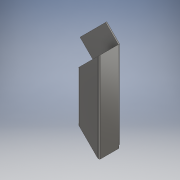
# Autodesk Inventor part: TestPlate
Saved by Autodesk Inventor 2018 (Build 220112000, 112)
## iProperties
Created: 2018-02-27
Part Number: TestPlate
Material: Steel, Mild
Document SubType Name: Modeling
Designer: P136265
Density: 7.85 g/cm^3
Appearance: Semi-Polished
Mass: 466.656 g
Surface Area: 399.113 cm^2
Volume: 59.4467 cm^3
Author: P136265
Autodesk Inventor part; units mm, degrees
ref_plane "YZ Plane" through (0, 0, 0) normal (1, 0, 0) x (0, 1, 0)
ref_plane "XZ Plane" through (0, 0, 0) normal (0, 1, 0) x (-1, 0, 0)
ref_plane "XY Plane" through (0, 0, 0) normal (0, 0, 1) x (1, 0, 0)
sketch "Sketch1" plane through (0, 0, 0) normal (0, 0, 1) x (1, 0, 0)
  line L0 (-15, -17.5) -> (15, -17.5)
  line L1 (17.5, -15) -> (17.5, 15)
  line L2 (15, 17.5) -> (-15, 17.5)
  line L3 (-17.5, 15) -> (-17.5, -15)
  line L4 (-17.5, -17.5) -> (17.5, 17.5) construction
  line L5 (17.5, -17.5) -> (-17.5, 17.5) construction
  line L6 (-14.5, -14.5) -> (14.5, -14.5)
  line L7 (14.5, -14.5) -> (14.5, 14.5)
  line L8 (14.5, 14.5) -> (-14.5, 14.5)
  line L9 (-14.5, 14.5) -> (-14.5, -14.5)
  line L10 (-14.5, -14.5) -> (14.5, 14.5) construction
  line L11 (14.5, -14.5) -> (-14.5, 14.5) construction
  arc A0 (-15, 17.5) -> (-17.5, 15) centre (-15, 15) ccw
  arc A1 (17.5, 15) -> (15, 17.5) centre (15, 15) ccw
  arc A2 (15, -17.5) -> (17.5, -15) centre (15, -15) ccw
  arc A3 (-17.5, -15) -> (-15, -17.5) centre (-15, -15) ccw
  point P0 (0, 0)
  dimension "d0" = 35
  dimension "d1" = 35
  dimension "d2" = 29
  dimension "d3" = 29
  dimension "d4" = 2.5
  constraints: 24 end point, 8 point on circle, 8 point on line, 8 tangent, 4 centre point, 4 midpoint, 4 parallel, 3 equal radius, 2 horizontal, 2 perpendicular
  measures "d0" distance of L5.end L4.end
  measures "d1" distance of L4.end L5.start
  measures "d2" distance of L8.end L7.end
  measures "d3" distance of L7.end L6.end
  measures "d4" radius of A0
extrude "Extrusion1" add sketch "Sketch1" along normal blind 150
sketch "Sketch2" plane through (-15, 17.5, 0) normal (0, 1, 0) x (1, 0, 0)
  line L0 (30, 0) -> (0, 0) construction
  line L1 (0, 0) -> (0, -150) construction
  line L2 (30, -150) -> (0, -150) construction
  line L3 (30, 0) -> (30, -150) construction
  line L4 (-2.5, 0) -> (-2.5, -150) construction
  line L5 (32.5, 0) -> (32.5, -150) construction
  line L6 (-7.5, 0) -> (32.5, 0)
  line L7 (-7.5, 0) -> (-7.5, -40)
  line L8 (-7.5, -40) -> (32.5, 0)
  line L9 (0, 0) -> (0, -150) construction
  line L10 (0, -75) -> (29.5, -75) construction
  line L11 (29.5, 0) -> (29.5, -150) construction
  line L12 (-7.5, -150) -> (32.5, -150)
  line L13 (-7.5, -150) -> (-7.5, -110)
  line L14 (-7.5, -110) -> (32.5, -150)
  point P0 (15, 0)
  dimension "d7" = 40
  dimension "d8" = 40
  constraints: 14 end point, 2 midpoint, 2 symmetric about line, 1 horizontal, 1 vertical
  measures "d7" distance of L6.start L5.start
  measures "d8" distance of L6.start L7.end
extrude "Extrusion2" cut sketch "Sketch2" against normal blind 100
sketch "Sketch5" plane through (15, 17.5, 147.5) normal (0, 1, 0) x (1, 0, 0)
  line L0 (-30, 30) -> (0, 0) construction
  line L1 (2.5, -2.5) -> (0, 0) projected
  line L2 (0, 0) -> (-42.4264, 42.4264) construction
  line L3 (-42.4264, 42.4264) -> (-63.6396, 21.2132)
  line L4 (-63.6396, 21.2132) -> (-21.2132, -21.2132)
  line L5 (-21.2132, -21.2132) -> (0, 0)
  line L6 (0, 145) -> (-30, 115) construction
  line L7 (0, 145) -> (2.5, 147.5) projected
  line L8 (0, 0) -> (0, 145)
  line L9 (-30, 115) -> (-30, 30) construction
  line L10 (-30, 72.5) -> (-0.5, 72.5) construction
  line L11 (-0.5, 144.5) -> (-0.5, 0.5) construction
  line L12 (0, 145) -> (-42.4264, 102.5736) construction
  line L13 (-42.4264, 102.5736) -> (-63.6396, 123.7868)
  line L14 (-63.6396, 123.7868) -> (-21.2132, 166.2132)
  line L15 (-21.2132, 166.2132) -> (0, 145)
  line L16 (-42.4264, 102.5736) -> (-42.4264, 42.4264)
  point P0 (-15, 147.5)
  dimension "d18" = 60
  dimension "d19" = 30
  constraints: 22 end point, 3 perpendicular, 3 symmetric about line, 2 midpoint, 2 vertical, 1 point on line
  measures "d18" distance of L0.end L2.end
  measures "d19" distance of L2.end L3.end
extrude "Extrusion5" add sketch "Sketch5" along normal blind 2
body "Solid1"
